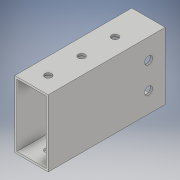
# Autodesk Inventor part: Bumper attachment frame
Saved by Autodesk Inventor 2018 (Build 220112000, 112)
## iProperties
Created: 2019-01-29
Part Number: Bumper attachment frame
Material: Generic
Document SubType Name: Modeling
Designer: maste
Density: 1 g/cm^3
Appearance: Default
Author: maste
Autodesk Inventor part; units mm, degrees
ref_plane "YZ Plane" through (0, 0, 0) normal (1, 0, 0) x (0, 1, 0)
ref_plane "XZ Plane" through (0, 0, 0) normal (0, 1, 0) x (-1, 0, 0)
ref_plane "XY Plane" through (0, 0, 0) normal (0, 0, 1) x (1, 0, 0)
sketch "Sketch1" plane through (0, 0, 0) normal (0, 0, 1) x (1, 0, 0)
  line L0 (0, 0) -> (25.4, 0)
  line L1 (25.4, 0) -> (25.4, 50.8)
  line L2 (25.4, 50.8) -> (0, 50.8)
  line L3 (0, 50.8) -> (0, 0)
  line L4 (1.5875, 49.2125) -> (23.8125, 49.2125)
  line L5 (23.8125, 49.2125) -> (23.8125, 1.5875)
  line L6 (23.8125, 1.5875) -> (1.5875, 1.5875)
  line L7 (1.5875, 1.5875) -> (1.5875, 49.2125)
  dimension "d0" = 25.4
  dimension "d1" = 50.8
  dimension "d2" = 1.5875
  constraints: 16 end point, 4 parallel, 2 perpendicular, 1 horizontal, 3 other
  measures "d0" distance of L2.end L1.end
  measures "d1" distance of L1.end L0.end
  measures "d2" distance between parallel lines of L2 L4
extrude "Extrusion1" add sketch "Sketch1" along normal blind 88.9
sketch "Sketch2" plane through (25.4, 0, 0) normal (1, 0, 0) x (0, 0, -1)
  line L0 (0, 0) -> (0, 50.8) construction
  line L1 (0, 50.8) -> (-12.7, 50.8) construction
  line L2 (0, 50.8) -> (-88.9, 50.8) construction
  line L3 (0, 25.4) -> (-12.7, 25.4) construction
  line L4 (-12.7, 25.4) -> (-12.7, 35.4) construction
  line L5 (-12.7, 35.4) -> (-12.7, 15.4) construction
  circle A0 centre (-12.7, 35.4) radius 3
  circle A1 centre (-12.7, 15.4) radius 3
  dimension "d5" = 12.7
  dimension "d6" = 10
  dimension "d7" = 20
  dimension "d8" = 6
  constraints: 8 end point, 2 centre point, 2 coincident, 2 point on line, 1 horizontal, 1 midpoint, 1 perpendicular
  measures "d5" distance of L0.end L1.end
  measures "d6" distance of L3.end L4.end
  measures "d7" distance of L4.end L5.end
  measures "d8" diameter of A0
extrude "Extrusion2" cut sketch "Sketch2" against normal blind 88.9
sketch "Sketch3" plane through (0, 50.8, 0) normal (0, 1, 0) x (1, 0, 0)
  line L0 (1.5875, -88.9) -> (23.8125, -88.9) construction
  line L1 (12.7, -88.9) -> (12.7, -76.2) construction
  line L2 (12.7, -76.2) -> (12.7, -50.8) construction
  line L3 (12.7, -50.8) -> (12.7, -25.4) construction
  circle A0 centre (12.7, -76.2) radius 2.5797
  circle A1 centre (12.7, -50.8) radius 2.5797
  circle A2 centre (12.7, -25.4) radius 2.5797
  point P0 (0, 0)
  dimension "d11" = 12.7
  dimension "d12" = 25.4
  dimension "d13" = 25.4
  dimension "d14" = 5.1594
  constraints: 6 end point, 3 centre point, 3 coincident, 2 point on line, 1 midpoint, 1 vertical
  measures "d11" distance of L1.start L1.end
  measures "d12" distance of L1.end L2.end
  measures "d13" distance of L2.end L3.end
  measures "d14" diameter of A0
extrude "Extrusion3" cut sketch "Sketch3" against normal blind 88.9
body "Solid1"
